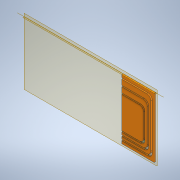
# Autodesk Inventor part: primary_coil_0R2
Saved by Autodesk Inventor 2021 (Build 250183000, 183)
## iProperties
Created: 2021-01-20
Part Number: primary_coil_0R2
Material: Generic
Document SubType Name: Modeling
Designer: phamv
Density: 1 g/cm^3
Appearance: Default
Author: phamv
Autodesk Inventor part; units mm, degrees
ref_plane "YZ Plane" through (0, 0, 0) normal (1, 0, 0) x (0, 1, 0)
sketch "Sketch1" plane through (0, 0, 0) normal (0, 0, 1) x (1, 0, 0)
  line L0 (0, -9.3) -> (385, -9.3)
  line L1 (400, -24.3) -> (400, -185)
  line L2 (385, -200) -> (-400, -200)
  line L3 (-400, -200) -> (-400, -32.4)
  line L4 (0, -9.3) -> (0, -13.8)
  line L5 (0, -13.8) -> (380.5, -13.8)
  line L6 (395.5, -28.8) -> (395.5, -180.5)
  line L7 (380.5, -195.5) -> (-395.5, -195.5)
  line L8 (-400, -32.4) -> (372.25, -32.4)
  line L9 (387.25, -47.4) -> (387.25, -172.25)
  line L10 (372.25, -187.25) -> (-387.25, -187.25)
  line L11 (-395.5, -195.5) -> (-395.5, -36.9)
  line L12 (-395.5, -36.9) -> (367.75, -36.9)
  line L13 (382.75, -51.9) -> (382.75, -167.75)
  line L14 (367.75, -182.75) -> (-382.75, -182.75)
  line L15 (-382.75, -182.75) -> (-382.75, -60)
  line L16 (-387.25, -187.25) -> (-387.25, -55.5)
  line L17 (-387.25, -55.5) -> (359.5, -55.5)
  line L18 (374.5, -70.5) -> (374.5, -159.5)
  line L19 (-382.75, -60) -> (355, -60)
  line L20 (370, -75) -> (370, -155)
  line L21 (-561.3296, 0) -> (567.9776, 0) projected
  line L22 (355, -170) -> (-374.5, -170)
  line L23 (359.5, -174.5) -> (-374.5, -174.5)
  line L24 (-374.5, -174.5) -> (-374.5, -170)
  arc A0 (400, -24.3) -> (385, -9.3) centre (385, -24.3) ccw
  arc A1 (395.5, -28.8) -> (380.5, -13.8) centre (380.5, -28.8) ccw
  arc A2 (387.25, -47.4) -> (372.25, -32.4) centre (372.25, -47.4) ccw
  arc A3 (382.75, -51.9) -> (367.75, -36.9) centre (367.75, -51.9) ccw
  arc A4 (374.5, -70.5) -> (359.5, -55.5) centre (359.5, -70.5) ccw
  arc A5 (370, -75) -> (355, -60) centre (355, -75) ccw
  arc A6 (355, -170) -> (370, -155) centre (355, -155) ccw
  arc A7 (359.5, -174.5) -> (374.5, -159.5) centre (359.5, -159.5) ccw
  arc A8 (367.75, -182.75) -> (382.75, -167.75) centre (367.75, -167.75) ccw
  arc A9 (372.25, -187.25) -> (387.25, -172.25) centre (372.25, -172.25) ccw
  arc A10 (380.5, -195.5) -> (395.5, -180.5) centre (380.5, -180.5) ccw
  arc A11 (385, -200) -> (400, -185) centre (385, -185) ccw
  line L25 (406.648, 0) -> (293.548, 0)
  line L26 (293.548, 0) -> (293.548, -209.55)
  line L27 (293.548, -209.55) -> (406.648, -209.55)
  line L28 (406.648, -209.55) -> (406.648, 0)
  point P0 (0, 0)
  point P1 (400, -9.3)
  point P2 (400, -200)
  point P3 (395.5, -13.8)
  point P4 (395.5, -195.5)
  point P5 (387.25, -32.4)
  point P6 (387.25, -187.25)
  point P7 (382.75, -36.9)
  point P8 (382.75, -182.75)
  point P9 (374.5, -55.5)
  point P10 (374.5, -174.5)
  point P11 (370, -60)
  point P12 (370, -170)
  point P13 (0, 0)
  point P14 (293.548, -200)
  point P15 (293.548, 0)
  point P16 (293.548, -9.3)
  point P17 (293.548, -13.8)
  point P18 (293.548, -32.4)
  point P19 (293.548, -187.25)
  point P20 (293.548, -195.5)
  point P21 (293.548, -36.9)
  point P22 (293.548, -55.5)
  point P23 (293.548, -174.5)
  point P24 (293.548, -182.75)
  point P25 (293.548, -60)
  point P26 (293.548, -170)
  dimension "d1" = 4.5
  dimension "d2" = 4.5
  dimension "d3" = 4.5
  dimension "d4" = 9.3
  dimension "d5" = 800
  dimension "d6" = 400
  dimension "d7" = 4.5
  dimension "d8" = 4.5
  dimension "d9" = 8.25
  dimension "d10" = 4.5
  dimension "d11" = 18.6
  dimension "d12" = 4.5
  dimension "d13" = 8.25
  dimension "d14" = 4.5
  dimension "d15" = 4.5
  dimension "d16" = 4.5
  dimension "d17" = 8.25
  dimension "d19" = 18.6
  dimension "d20" = 8.25
  dimension "d82" = 200
  dimension "d88" = 4.5
  dimension "d89" = 8.25
  dimension "d90" = 8.25
  dimension "d91" = 15
  dimension "d100" = 113.1
  dimension "d101" = 209.55
  constraints: 56 end point, 25 point on line, 24 point on circle, 24 tangent, 16 perpendicular, 12 centre point, 11 equal radius, 5 horizontal, 4 parallel, 3 vertical, 1 coincident
  measures "d1" distance between parallel lines of L5 L0
  measures "d2" distance between parallel lines of L6 L1
  measures "d3" distance between parallel lines of L2 L7
  measures "d4" distance from line of L21 L0.start
  measures "d5" distance between parallel lines of L3 L1
  measures "d6" distance from line of point (0, 0) L1
  measures "d7" distance between parallel lines of L3 L11
  measures "d8" distance between parallel lines of L13 L9
  measures "d9" distance between parallel lines of L9 L6
  measures "d10" distance between parallel lines of L8 L12
  measures "d11" distance between parallel lines of L8 L5
  measures "d12" distance between parallel lines of L10 L14
  measures "d13" distance between parallel lines of L7 L10
  measures "d14" distance between parallel lines of L16 L15
  measures "d15" distance between parallel lines of L17 L19
  measures "d16" distance between parallel lines of L20 L18
  measures "d17" distance between parallel lines of L18 L13
  measures "d19" distance between parallel lines of L17 L12
  measures "d20" distance between parallel lines of L11 L16
  measures "d82" distance between parallel lines of L2 L21
  measures "d88" distance between parallel lines of L23 L22
  measures "d89" distance between parallel lines of L14 L23
  measures "d90" distance between parallel lines of L15 L24
  measures "d91" radius of A0
  measures "d100" distance between parallel lines of L26 L28
  measures "d101" distance between parallel lines of L21 L27
extrude "Extrusion1" add sketch "Sketch1" along normal blind 4.5 contours L26 L21 L28 L27 L2 A11 L1 A0 L0 | L5 A1 L6 A10 L7 L26 L10 A9 L9 A2 L8 | L12 A3 L13 A8 L14 L26 L23 A7 L18 A4 L17 | L19 A5 L20 A6 L22 L26
ref_plane "basePlane" through (0, 0, 0) normal (0, 0, -1) x (-1, 0, 0)
sketch "Sketch5" plane through (0, 0, 0) normal (0, 0, -1) x (-1, 0, 0)
  line L0 (-406.648, 0) -> (-293.548, 0) projected
  line L1 (-406.648, -209.55) -> (-406.648, 0) projected
  line L2 (-293.548, 0) -> (-406.648, 0)
  line L3 (-406.648, 0) -> (-406.648, -209.55)
  line L4 (-406.648, -209.55) -> (-293.548, -209.55)
  line L5 (-293.548, -209.55) -> (-293.548, 0)
  point P0 (0, 0)
  constraints: 8 end point, 2 parallel, 1 horizontal, 1 perpendicular
extrude "Extrusion5" add sketch "Sketch5" along normal blind 0.45
equation "\"d1\" = wire_diameter"
equation "\"d2\" = wire_diameter"
equation "\"d3\" = wire_diameter"
equation "\"d4\" = 0.5 * distance_between_wires"
equation "\"d5\" = track_length"
equation "\"d6\" = 0.5 * track_length"
equation "\"d7\" = wire_diameter"
equation "\"d8\" = wire_diameter"
equation "\"d9\" = distance_between_wires_edge"
equation "\"d10\" = wire_diameter"
equation "\"d11\" = distance_between_wires"
equation "\"d12\" = wire_diameter"
equation "\"d13\" = distance_between_wires_edge"
equation "\"d14\" = wire_diameter"
equation "\"d15\" = wire_diameter"
equation "\"d16\" = wire_diameter"
equation "\"d17\" = distance_between_wires_edge"
equation "\"d19\" = distance_between_wires"
equation "\"d20\" = distance_between_wires_edge"
equation "\"d82\" = 0.5 * track_width"
equation "\"d22\" = wire_diameter"
equation "\"track_length\" = 800"
equation "\"wire_diameter\" = 4.5"
equation "\"distance_between_wires\" = -1.2 * wire_diameter + 0.2 * parameter_6"
equation "\"distance_between_wires_edge\" = 8.25"
equation "\"bend_radius\" = 15"
equation "\"track_width\" = 400"
equation "\"parameter_6\" = 120"
body "Solid1"
